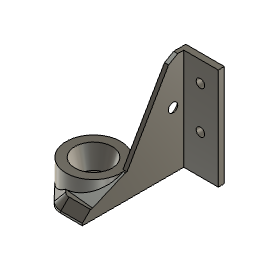
Hinge_Front_Left_Top_and_Rear_Right_Bottom (Autodesk Fusion 360 design; units mm, degrees)
Autodesk Fusion 360 part; units mm, degrees
note: some values were not read from the file. Chosen so that the rebuilt part matches the saved one: which face or edge a step refers to; which pieces of a blend or face edit are solid.
sketch "Skizze1" plane through (0, 0, 0) normal (0, 0, 1) x (1, 0, 0)
  line L0 (0, 0) -> (19, 0)
  line L1 (19, 0) -> (19, 6)
  line L2 (19, 6) -> (0, 6)
  line L3 (0, 6) -> (0, 0)
  line L4 (0, 0) -> (2, 0)
  line L5 (2, 0) -> (2, -50)
  line L6 (2, -50) -> (-12, -50)
  line L7 (-12, -50) -> (-12, -30)
  line L8 (-12, -30) -> (-12.5, -30)
  circle A0 centre (-12.5, -30) radius 13.5
  line L9 (-12, -50) -> (-22.2324, -39.3558)
  line L10 (0, 6) -> (-22.8574, -21.3412)
  circle A1 centre (-12.5, -30) radius 6.2
  dimension "d1" = 6
  dimension "d2" = 19
  dimension "d3" = 2
  dimension "d4" = 50
  dimension "d5" = 14
  dimension "d6" = 20
  dimension "d7" = 0.5
  dimension "d8" = 27
  dimension "d9" = 12.4
  constraint horizontal L0
  constraint vertical L1
  constraint horizontal L2
  constraint vertical L3
  constraint coincident L0.start L3.end
  constraint perpendicular L3 L4
  constraint perpendicular L0 L5
  constraint perpendicular L5 L6
  constraint perpendicular L6 L7
  constraint horizontal L8
  constraint coincident L8.end A0.centre
  constraint coincident A0 L9.end
  constraint tangent A0 L9
  constraint coincident A0 L10.end
  constraint tangent A0 L10
  constraint concentric A0 A1
  measures "d1" distance of L0.start L2.end
  measures "d2" distance of L0.start L0.end
  measures "d3" distance of L0.start L4.end
  measures "d4" distance of L4.end L5.end
  measures "d5" distance of L5.end L6.end
  measures "d6" distance of L6.end L7.end
  measures "d7" distance of L7.end L8.end
  measures "d8" diameter of A0
  measures "d9" diameter of A1
extrude "Extrusion1" add sketch "Skizze1" along normal blind 2 contours A1
extrude "Extrusion2" add sketch "Skizze1" along normal blind 12 contours A0
chamfer "Fase1" distance 3 distance2 10 1 edges at (-18.2804, -27.758, 12) measured on face at (-1.5067, -29.0213, 12)
extrude "Extrusion3" add sketch "Skizze1" along normal blind 5 contours L0 L1 L2 L3 L4 | L0 L3 L4 L5 L6 L7 A0 L10 | L7 A0 L9
sketch "Skizze2" plane through (0, 0, 5) normal (0, 0, 1) x (-1, 0, 0)
  line L0 (-2, 0) -> (-19, 0)
  line L1 (-19, 0) -> (-19, -6)
  line L2 (-19, -6) -> (0, -6)
  line L3 (0, -6) -> (22.8574, 21.3412)
  arc A0 (22.2324, 39.3558) -> (22.8574, 21.3412) centre (12.5, 30) ccw
  line L4 (22.2324, 39.3558) -> (12, 50)
  line L5 (12, 50) -> (-2, 50)
  line L6 (-2, 50) -> (-2, 0)
  line L7 (-2, 0) -> (0, 0)
  line L8 (0, 0) -> (0, -6)
  line L9 (-2, 30.0242) -> (-1, 30.0242)
  line L10 (1.1977, 22.617) -> (0, 20)
  line L11 (0, 20) -> (0, 0)
  line L12 (0, 15) -> (12.9222, 16.5066)
  line L13 (-2, 44.95) -> (12.4619, 43.4999)
  constraint coincident L0.start L6.end
  constraint coincident L7.end L8.start
  constraint coincident L2.end L3.start
  constraint coincident L6 L9.start
  constraint coincident A0 L9.end
  constraint perpendicular L6 L9
  constraint coincident A0 L10.start
  constraint perpendicular L7 L11
  constraint coincident L11 L12.start
  constraint coincident A0 L12.end
  constraint coincident L6 L13.start
  constraint coincident A0 L13.end
extrude "Extrusion4" add sketch "Skizze2" along normal blind 45 contours L0 L1 L2 L7 L8
extrude "Extrusion5" add sketch "Skizze2" along normal blind 7 contours A0 L6 L7 L9 L10 L11 | A0 L10 L11 L12
sketch "Skizze3" plane through (0, 0, 12) normal (0, 0, 1) x (-1, 0, 0)
  arc A0 (12.9222, 16.5066) -> (-1, 30.0242) centre (12.5, 30) ccw
  line L0 (-1, 30.0242) -> (-2, 30.0242)
  line L1 (-2, 30.0242) -> (-2, 0)
  line L2 (-2, 0) -> (0, 0)
  line L3 (0, 0) -> (0, 15)
  line L4 (0, 15) -> (12.9222, 16.5066)
  circle A1 centre (12.5, 30) radius 9.2
  line L5 (0, 15) -> (0, 28)
  line L6 (0, 28) -> (-2, 28)
  constraint coincident L3.end L4.start
  constraint parallel L3 L5
  constraint coincident L1 L6.end
extrude "Extrusion6" add sketch "Skizze3" along normal blind 38 contours L1 L2 L3 L5 L6
chamfer "Fase2" distance 22 distance2 38 1 edges at (1, -28, 50) measured on face at (7, 4, 50)
extrude "Extrusion7" add sketch "Skizze2" along normal blind 7 contours A0 L6 L9 L13
chamfer "Fase3" distance 16 distance2 7 1 edges at (-5.231, -44.225, 12) measured on face at (-6.1207, -42.1389, 12)
chamfer "Fase4" distance 8 distance2 7 1 edges at (-6.4611, -15.7533, 12) measured on face at (-7.3538, -17.6477, 12)
fillet "Abrundung1" radius 8 1 edges at (-12, -50, 2.5)
chamfer "Fase5" distance 3 angle 45 1 edges at (1, -6.0044, 50)
sketch "Skizze4" plane through (0, 6, 0) normal (0, 1, 0) x (-1, 0, 0)
  line L0 (-19, 0) -> (0, 0)
  line L1 (0, 0) -> (0, 5)
  line L2 (0, 5) -> (0, 50)
  line L3 (0, 50) -> (-19, 50)
  line L4 (-19, 50) -> (-19, 0)
  line L5 (-19, 50) -> (-10.2, 50)
  line L6 (-10.2, 50) -> (-10.2, 39.9)
  line L7 (-10.2, 39.9) -> (-19, 39.9)
  line L8 (-19, 39.9) -> (-19, 50)
  line L9 (-19, 0) -> (-10.2, 0)
  line L10 (-10.2, 0) -> (-10.2, 19.1)
  line L11 (-10.2, 19.1) -> (-19, 19.1)
  line L12 (-19, 19.1) -> (-19, 0)
  dimension "d34" = 10.1
  dimension "d35" = 8.8
  dimension "d36" = 19.1
  dimension "d37" = 8.8
  constraint horizontal L5
  constraint vertical L6
  constraint horizontal L7
  constraint vertical L8
  constraint coincident L3.end L4.start
  constraint horizontal L9
  constraint vertical L10
  constraint horizontal L11
  constraint vertical L12
  constraint coincident L0.start L4.end
  measures "d34" distance of L3.end L7.end
  measures "d35" distance of L3.end L5.end
  measures "d36" distance of L0.start L11.end
  measures "d37" distance of L0.start L9.end
hole "Bohrung1" at (10.2, 6, 39.9) at (10.2, 6, 19.1) direction (0, -1, 0) diameter 4.2 depth 13 tip angle 180 countersink diameter 8.6 countersink angle 90
sketch "Skizze5" plane through (0, 0, 0) normal (-1, 0, 0) x (0, -1, 0)
  line L0 (7.5031, 47.4037) -> (3, 50)
  line L1 (3, 50) -> (-6, 50)
  line L2 (-6, 50) -> (-6, 5)
  line L3 (-6, 5) -> (15, 5)
  line L4 (15, 5) -> (23.0542, 12)
  line L5 (23.0542, 12) -> (28, 12)
  line L6 (28, 12) -> (7.5031, 47.4037)
  line L7 (-6, 5) -> (5.3, 5)
  line L8 (5.3, 5) -> (5.3, 28.1)
  line L9 (5.3, 28.1) -> (-6, 28.1)
  line L10 (-6, 28.1) -> (-6, 5)
  dimension "d46" = 11.3
  dimension "d47" = 23.1
  constraint horizontal L7
  constraint vertical L8
  constraint horizontal L9
  constraint vertical L10
  constraint coincident L2.end L3.start
  measures "d46" distance of L2.end L7.end
  measures "d47" distance of L2.end L9.end
hole "Bohrung2" at (0, -5.3, 28.1) direction (1, 0, 0) diameter 4.2 depth 13 tip angle 180 countersink diameter 8.6 countersink angle 90
chamfer "Fase6" distance 3 angle 45 3 edges at (19, 6, 25) (9.5, 6, 50) (0, 6, 27.5)
chamfer "Fase7" distance 4 angle 45 1 edges at (-11.4287, -7.6706, 5)
chamfer "Fase8" distance 4 angle 45 3 edges at (-18.2966, -43.45, 5) (-11.7277, -49.3605, 5) (-3.2967, -50, 5)
